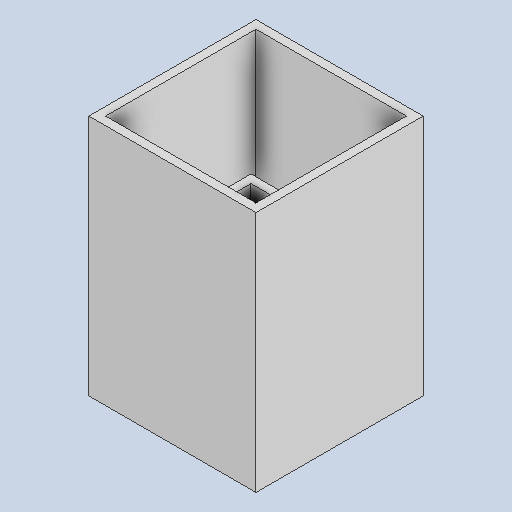
# Autodesk Inventor part: Część2
Saved by Autodesk Inventor 2022 (Build 260153000, 153)
## iProperties
Created: 2022-07-14
Part Number: Część2
Material: Ogólny
Document SubType Name: Sheet Metal
Designer: kosak
Density: 1 g/cm^3
Appearance: Domyślna
Sheet Metal Rule: Domyślny
Author: kosak
## iProperties of the stored document Część2_Drukowanie 3D.ipt
Created: 2022-07-14
Part Number: Część2_Drukowanie 3D
Material: Ogólny
Document SubType Name: Modeling
Designer: kosak
Density: 1 g/cm^3
Appearance: Domyślna
Author: kosak
Autodesk Inventor part; units mm, degrees
ref_plane "YZ Plane" through (0, 0, 0) normal (1, 0, 0) x (0, 1, 0)
ref_plane "XZ Plane" through (0, 0, 0) normal (0, 1, 0) x (-1, 0, 0)
ref_plane "XY Plane" through (0, 0, 0) normal (0, 0, 1) x (1, 0, 0)
sketch "Szkic1" plane through (0, 0, 0) normal (0, 1, 0) x (-1, 0, 0)
  line L0 (100, 100) -> (-100, 100)
  line L1 (-100, 100) -> (-100, -100)
  line L2 (-100, -100) -> (100, -100)
  line L3 (100, -100) -> (100, 100)
  point P0 (0, 0)
  constraints: 8 end point, 2 parallel, 1 horizontal, 1 perpendicular
extrude "Wyciągnięcie proste1" add sketch "Szkic1" against normal blind 290
sketch "Szkic2" plane through (0, -290, 0) normal (0, -1, 0) x (1, 0, 0)
  line L0 (100, -100) -> (100, 100) projected
  line L1 (100, 100) -> (-100, 100) projected
  line L2 (-100, 100) -> (-100, -100) projected
  line L3 (-100, -100) -> (100, -100) projected
  line L4 (-90, 90) -> (90, 90)
  line L5 (90, 90) -> (90, -90)
  line L6 (90, -90) -> (-90, -90)
  line L7 (-90, -90) -> (-90, 90)
  point P0 (0, 0)
  dimension "d6" = 10
  constraints: 8 end point, 3 other
  measures "d6" distance between parallel lines of L1 L4
extrude "Wyciągnięcie proste2" cut sketch "Szkic2" against normal blind 115.5 contours L4 L5 L6 L7
sketch "Szkic5" plane through (0, 0, 0) normal (0, 1, 0) x (1, 0, 0)
  line L0 (100, -100) -> (100, 100) projected
  line L1 (100, 100) -> (-100, 100) projected
  line L2 (-100, 100) -> (-100, -100) projected
  line L3 (-100, -100) -> (100, -100) projected
  line L4 (-90, 90) -> (90, 90)
  line L5 (90, 90) -> (90, -90)
  line L6 (90, -90) -> (-90, -90)
  line L7 (-90, -90) -> (-90, 90)
  point P0 (0, 0)
  dimension "d14" = 10
  constraints: 8 end point, 3 other
  measures "d14" distance between parallel lines of L1 L4
sketch "Szkic11" plane through (0, -290, 0) normal (0, -1, 0) x (1, 0, 0)
  circle A0 centre (94.2929, 94.2929) radius 3 projected
  circle A1 centre (94.2929, 94.2929) radius 4
  line L0 (100, 100) -> (-100, 100) projected
  line L1 (0, 100) -> (0, 94.6465)
  line L2 (100, -100) -> (100, 100) projected
  line L3 (100, 0) -> (94.6465, 0)
  circle A2 centre (-94.2929, 94.2929) radius 4
  circle A3 centre (94.2929, -94.2929) radius 4
  circle A4 centre (-94.2929, -94.2929) radius 4
  point P0 (0, 0)
  dimension "d35" = 8
  constraints: 4 centre point, 4 end point, 3 symmetric about line, 2 midpoint, 1 coincident, 1 horizontal, 1 vertical, 3 other
  measures "d35" diameter of A1
extrude "Wyciągnięcie proste9" cut sketch "Szkic11" against normal blind 2 contours A0 | A1 | A2 | A3 | A4
extrude "Wyciągnięcie proste10" cut sketch "Szkic5" against normal blind 164.5 contours L4 L5 L6 L7
sketch "Szkic12" plane through (-90, 0, 90) normal (1, 0, 0) x (0, 0, -1)
  line L0 (42.4083, -290.7928) -> (42.4083, -131.7928)
  line L1 (0, 0) -> (0, -164.5) projected
  line L2 (180, 0) -> (180, -164.5) projected
  line L3 (0, -136.7928) -> (180, -136.7928)
  line L4 (180, -136.7928) -> (180, -126.7928)
  line L5 (180, -126.7928) -> (0, -126.7928)
  line L6 (0, -126.7928) -> (0, -136.7928)
  point P0 (90, 0)
  dimension "d40" = 159
  dimension "d41" = 10
  constraints: 10 end point, 2 parallel, 2 point on line, 1 horizontal, 1 perpendicular, 1 vertical
  measures "d40" distance of L0.start L0.end
  measures "d41" distance of L4.end L3.end
extrude "Wyciągnięcie proste11" add sketch "Szkic12" along normal blind 85.5
sketch "Szkic13" plane through (-90, -126.7928, 90) normal (0, 1, 0) x (1, 0, 0)
  point P0 (90, 90)
sketch "Szkic14" plane through (-90, -126.7928, 90) normal (0, 1, 0) x (1, 0, 0)
  line L0 (85.5, 0) -> (95.5, 0)
  line L1 (95.5, 0) -> (95.5, 180)
  line L2 (95.5, 180) -> (85.5, 180)
  line L3 (85.5, 180) -> (85.5, 0)
  point P0 (90, 90)
  dimension "d44" = 10
  dimension "d45" = 180
  constraints: 8 end point, 2 parallel, 1 horizontal, 1 perpendicular
  measures "d44" distance of L2.end L1.end
  measures "d45" distance of L1.end L0.end
extrude "Wyciągnięcie proste12" add sketch "Szkic14" against normal through all
sketch "Szkic15" plane through (0, -174.5, 0) normal (0, -1, 0) x (1, 0, 0)
  line L0 (-90, 90) -> (90, 90) projected
  line L1 (-90, -90) -> (-4.5, -90) projected
  line L2 (-90, 90) -> (-4.5, 90)
  line L3 (-4.5, 90) -> (-4.5, -90)
  line L4 (-4.5, -90) -> (-90, -90)
  line L5 (-90, -90) -> (-90, 90)
  point P0 (0, 0)
  constraints: 8 end point, 2 parallel, 1 horizontal, 1 perpendicular
extrude "Wyciągnięcie proste13" cut sketch "Szkic15" against normal blind 10
sketch "Szkic17" plane through (-90, -126.7928, 90) normal (0, 1, 0) x (1, 0, 0)
  line L0 (0, 180) -> (23, 180)
  line L1 (23, 180) -> (23, 163)
  line L2 (23, 163) -> (0, 163)
  line L3 (0, 163) -> (0, 180)
  point P0 (90, 90)
  dimension "d54" = 23
  dimension "d55" = 17
  constraints: 8 end point, 2 parallel, 1 horizontal, 1 perpendicular
  measures "d54" distance of L1.end L2.end
  measures "d55" distance of L0.end L1.end
extrude "Wyciągnięcie proste15" cut sketch "Szkic17" against normal through all
sketch "Szkic18" plane through (5.5, -126.7928, 90) normal (0, 1, 0) x (1, 0, 0)
  line L0 (-72.5, 180) -> (-72.5, 163) projected
  line L1 (-95.5, 0) -> (-95.5, 163) projected
  line L2 (-95.5, 163) -> (-72.5, 163)
  line L3 (-72.5, 153) -> (-95.5, 153)
  line L4 (-95.5, 153) -> (-95.5, 163)
  line L5 (-72.5, 180) -> (-62.5, 180)
  line L6 (-62.5, 180) -> (-62.5, 153)
  line L7 (-62.5, 153) -> (-72.5, 153)
  line L8 (-72.5, 180) -> (-72.5, 163)
  point P0 (-5.5, 90)
  point P1 (-95.5, 153)
  dimension "d58" = 10
  dimension "d59" = 10
  constraints: 14 end point, 3 equal length, 2 horizontal, 1 perpendicular, 1 point on line
  measures "d58" distance of L2.end L3.start
  measures "d59" distance of L6.end L7.end
extrude "Wyciągnięcie proste16" add sketch "Szkic18" along normal blind 126.793
equation "\"PromieńGięcia\" = Grubość"
equation "\"SzerokośćGięciaPodcięcia\" = Grubość"
equation "\"GłębokośćGięciaPodcięcia\" = 0.5 * Grubość"
equation "\"RozmiarPodcięciaNarożnika\" = 4 * Grubość"
equation "\"MinimalnaPozostałość\" = 2 * Grubość"
equation "\"PromieńPrzejścia\" = PromieńGięcia"
equation "\"Rozmiar_promienia_Jacobiego\" = PromieńGięcia"
equation "\"Wielk_odstępu\" = Grubość"
equation "\"Grubość\" = 3.048"
